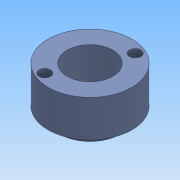
# Autodesk Inventor part: factory barrier adapter
Saved by Autodesk Inventor 2017 (Build 210142000, 142)
## iProperties
Part Number: factory barrier adapter
Material: Типовые
Document SubType Name: Modeling
Designer: Max
Mass: 2.66367 g
Surface Area: 19.448 cm^2
Volume: 2.66367 cm^3
Density: 1 g/cm^3
Appearance: Резина — синяя
Author: Max
Autodesk Inventor part; units mm, degrees
ref_plane "YZ Plane" through (0, 0, 0) normal (1, 0, 0) x (0, 1, 0)
ref_plane "XZ Plane" through (0, 0, 0) normal (0, 1, 0) x (-1, 0, 0)
ref_plane "XY Plane" through (0, 0, 0) normal (0, 0, 1) x (1, 0, 0)
sketch "Эскиз1" plane through (0, 0, 0) normal (0, 0, 1) x (1, 0, 0)
  circle A0 centre (0, 0) radius 7.95
  circle A1 centre (0, 0) radius 11
  circle A2 centre (0, 0) radius 6
  dimension "d0" = 15.9
  dimension "d1" = 22
  dimension "d2" = 12
  constraints: 3 centre point, 3 coincident
  measures "d0" diameter of A0
  measures "d1" diameter of A1
  measures "d2" diameter of A2
extrude "Выдавливание1" add sketch "Эскиз1" against normal blind 2.5 contours A0
extrude "Выдавливание2" add sketch "Эскиз1" along normal blind 9.7 contours A0 | A1
sketch "Эскиз2" plane through (0, 0, 0) normal (0, 0, -1) x (-1, 0, 0)
  circle A0 centre (3.6709, -8.2173) radius 1.5 projected
  circle A1 centre (-3.6709, 8.2173) radius 1.5 projected
  circle A2 centre (3.6709, -8.2173) radius 1.5
  circle A3 centre (-3.6709, 8.2173) radius 1.5
  point P0 (0, 0)
  dimension "d7" = 3
  dimension "d8" = 3
  constraints: 2 centre point, 2 coincident
  measures "d7" diameter of A2
  measures "d8" diameter of A3
extrude "Выдавливание3" cut sketch "Эскиз2" along normal mid plane 30
